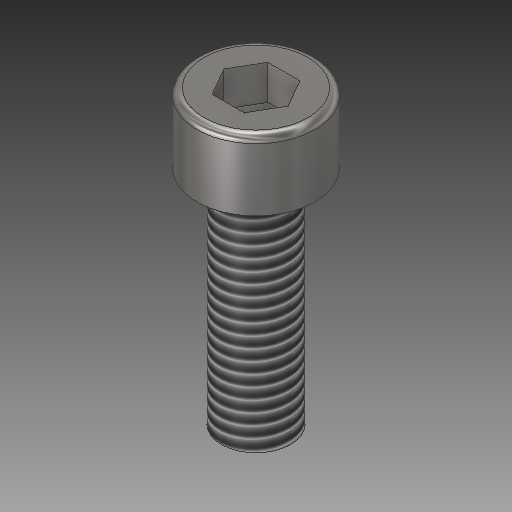
# Autodesk Inventor part: SSCF-M5-16-A4
Saved by Autodesk Inventor 2019 (Build 230136000, 136)
## iProperties
Created: 2018-04-23
Part Number: SSCF-M5-16-A4
Material: Stainless Steel AISI 317
Document SubType Name: Modeling
Designer: IEUser
Density: 8 g/cm^3
Appearance: Semi-Polished
Mass: 4.49479 g
Surface Area: 5.27134 cm^2
Volume: 0.561848 cm^3
Author: IEUser
Autodesk Inventor part; units mm, degrees
ref_plane "YZ Plane" through (0, 0, 0) normal (1, 0, 0) x (0, 1, 0)
ref_plane "XZ Plane" through (0, 0, 0) normal (0, 1, 0) x (-1, 0, 0)
ref_plane "XY Plane" through (0, 0, 0) normal (0, 0, 1) x (1, 0, 0)
sketch "Cap Cross Section" plane through (0, 0, 0) normal (0, 1, 0) x (-1, 0, 0)
  circle A0 centre (0, 0) radius 4.25
  dimension "d0" = 8.5
  constraints: 1 centre point, 1 coincident
  measures "d0" diameter of A0
extrude "Cap" add sketch "Cap Cross Section" along normal blind 5
sketch "Key Socket Cutout Outline" plane through (0, 5, 0) normal (0, 1, 0) x (1, 0, 0)
  line L0 (1.1547, 2) -> (2.3094, 0)
  line L1 (2.3094, 0) -> (1.1547, -2)
  line L2 (1.1547, -2) -> (-1.1547, -2)
  line L3 (-1.1547, -2) -> (-2.3094, 0)
  line L4 (-2.3094, 0) -> (-1.1547, 2)
  line L5 (-1.1547, 2) -> (1.1547, 2)
  point P0 (0, 0)
  point P1 (0, 0)
  dimension "d3" = 4
  constraints: 12 end point, 1 coincident, 1 horizontal, 13 other
  measures "d3" distance between parallel lines of L2 L5
extrude "Key Socket Cutout" cut sketch "Key Socket Cutout Outline" against normal blind 2.5
sketch "Body Cross Section" plane through (0, 0, 0) normal (0, -1, 0) x (1, 0, 0)
  circle A0 centre (0, 0) radius 2.5
  dimension "d6" = 5
  constraints: 1 centre point, 1 coincident
  measures "d6" diameter of A0
extrude "Body" add sketch "Body Cross Section" along normal blind 16
thread "Thread" size "M5x0.8" class "6g" standard "ANSI Metric M Profile" full length
fillet "Cap Fillet" radius 0.5 1 edges at (4.25, 5, 0)
body "Solid1"
